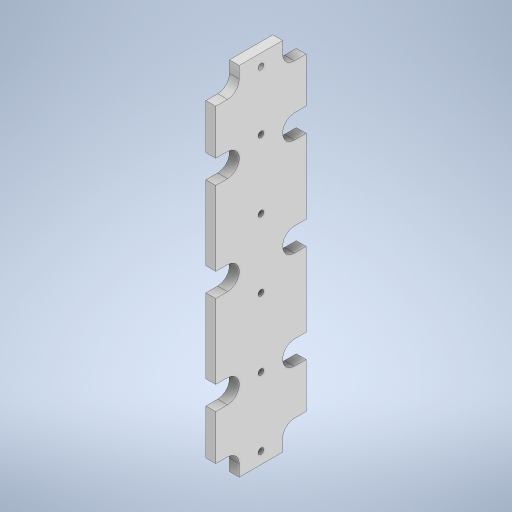
# Autodesk Inventor part: linrail_screw_spacer
Saved by Autodesk Inventor 2024 (Build 280153000, 153)
## iProperties
Created: 2025-12-26
Part Number: linrail_screw_spacer
Material: PET Plastic
Document SubType Name: Sheet Metal
Designer: schar
Density: 1.541 g/cm^3
Sheet Metal Rule: Default_mm
Appearance: Polycarbonate - Clear
Author: schar
Autodesk Inventor part; units mm, degrees
ref_plane "YZ Plane" through (0, 0, 0) normal (1, 0, 0) x (0, 1, 0)
ref_plane "XZ Plane" through (0, 0, 0) normal (0, 1, 0) x (-1, 0, 0)
ref_plane "Work Plane2" through (3, -200, 0) normal (1, 0, 0) x (0, 0, -1)
sketch "Sketch1" plane through (3, -200, 0) normal (1, 0, 0) x (0, 0, -1)
  circle A0 centre (10, 15) radius 2.5 projected
  circle A1 centre (10, 15) radius 6
  circle A2 centre (44.112, 15) radius 2.5 projected
  circle A3 centre (44.112, 15) radius 6
  circle A4 centre (44.112, 50) radius 2.5 projected
  circle A5 centre (44.112, 50) radius 6
  circle A6 centre (10, 50) radius 2.5 projected
  circle A7 centre (10, 50) radius 6
  circle A8 centre (10, 100) radius 2.5 projected
  circle A9 centre (10, 100) radius 6
  circle A10 centre (44.112, 100) radius 2.5 projected
  circle A11 centre (44.112, 100) radius 6
  circle A12 centre (10, 150) radius 2.5 projected
  circle A13 centre (10, 150) radius 6
  circle A14 centre (44.112, 150) radius 2.5 projected
  circle A15 centre (44.112, 150) radius 6
  circle A16 centre (10, 185) radius 2.5 projected
  circle A17 centre (10, 185) radius 6
  circle A18 centre (44.112, 185) radius 2.5 projected
  circle A19 centre (44.112, 185) radius 6
  circle A20 centre (27.056, 185) radius 1.5 projected
  circle A21 centre (27.056, 185) radius 1.5
  circle A22 centre (27.056, 155) radius 1.5 projected
  circle A23 centre (27.056, 155) radius 1.5
  circle A24 centre (27.056, 120) radius 1.5 projected
  circle A25 centre (27.056, 120) radius 1.5
  circle A26 centre (27.056, 85) radius 1.5 projected
  circle A27 centre (27.056, 85) radius 1.5
  circle A28 centre (27.056, 50) radius 1.5 projected
  circle A29 centre (27.056, 50) radius 1.5
  circle A30 centre (27.056, 15) radius 1.5 projected
  circle A31 centre (27.056, 15) radius 1.5
  line L0 (44.112, 9) -> (50.112, 9)
  line L1 (10, 9) -> (4, 9)
  line L2 (10, 191) -> (4, 191)
  line L3 (44.112, 191) -> (50.112, 191)
  line L4 (4, 191) -> (50.112, 191)
  line L5 (50.112, 191) -> (50.112, 9)
  line L6 (50.112, 9) -> (4, 9)
  line L7 (4, 9) -> (4, 191)
  line L8 (10, 56) -> (4, 56)
  line L9 (10, 44) -> (4, 44)
  line L10 (44.112, 56) -> (50.112, 56)
  line L11 (44.112, 44) -> (50.112, 44)
  line L12 (44.112, 21) -> (50.112, 21)
  line L13 (10, 21) -> (4, 21)
  line L14 (10, 94) -> (4, 94)
  line L15 (10, 106) -> (4, 106)
  line L16 (10, 144) -> (4, 144)
  line L17 (10, 156) -> (4, 156)
  line L18 (44.112, 156) -> (50.112, 156)
  line L19 (44.112, 144) -> (50.112, 144)
  line L20 (44.112, 179) -> (50.112, 179)
  line L21 (10, 179) -> (4, 179)
  line L22 (16, 185) -> (16, 191)
  line L23 (38.112, 185) -> (38.112, 191)
  line L24 (16, 15) -> (16, 9)
  line L25 (38.112, 15) -> (38.112, 9)
  line L26 (44.112, 106) -> (50.112, 106)
  line L27 (44.112, 94) -> (50.112, 94)
  point P0 (0, 200)
  point P1 (50.112, 100)
  dimension "d1" = 12
  dimension "d2" = 12
  dimension "d3" = 12
  dimension "d4" = 12
  dimension "d5" = 12
  dimension "d6" = 12
  dimension "d7" = 12
  dimension "d8" = 12
  dimension "d9" = 12
  dimension "d10" = 12
  constraints: 52 end point, 24 point on circle, 18 point on line, 16 centre point, 16 coincident, 15 horizontal, 10 tangent, 3 parallel, 2 perpendicular, 22 other
  measures "d1" diameter of A1
  measures "d2" diameter of A3
  measures "d3" diameter of A5
  measures "d4" diameter of A7
  measures "d5" diameter of A9
  measures "d6" diameter of A11
  measures "d7" diameter of A13
  measures "d8" diameter of A15
  measures "d9" diameter of A17
  measures "d10" diameter of A19
extrude "Extrusion1" add sketch "Sketch1" along normal blind 5 contours A1 L13 L7 L9 A7 L8 L14 A9 L15 L16 A13 L17 L21 A17 L22 L4 L23 A19 L20 L5 L18 A15 L19 L26 A11 L27 L10 A5 L11 L12 A3 L25 L6 L24
equation "\"BendRadius\" = Thickness"
equation "\"BendReliefWidth\" = Thickness"
equation "\"BendReliefDepth\" = 0.5 * Thickness"
equation "\"CornerReliefSize\" = 4 * Thickness"
equation "\"MinimumRemnant\" = 2 * Thickness"
equation "\"TransitionRadius\" = BendRadius"
equation "\"JacobiRadiusSize\" = BendRadius"
equation "\"GapSize\" = Thickness"
equation "\"Thickness\" = 0.5"
body "Solid1"
